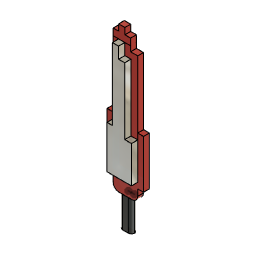
épée (Autodesk Fusion 360 design; units mm, degrees)
Autodesk Fusion 360 part; units mm, degrees
note: some values were not read from the file. Chosen so that the rebuilt part matches the saved one: which pieces of a blend or face edit are solid.
sketch "Esquisse1" plane through (0, 0, 0) normal (0, 0, 1) x (1, 0, 0)
  line L0 (304.8539, -213.5001) -> (-279.1145, -213.5001)
  line L1 (-279.1145, -213.5001) -> (-279.1145, 213.0938)
  line L2 (-279.1145, 213.0938) -> (304.8539, 213.0938)
  line L3 (304.8539, 213.0938) -> (304.8539, -213.5001)
  line L4 (443.4227, -65.0335) -> (-425, -65.0335)
  line L5 (-425, -65.0335) -> (-425, 75)
  line L6 (-425, 75) -> (443.4227, 75)
  line L7 (443.4227, 75) -> (443.4227, -65.0335)
  constraint horizontal L0
  constraint vertical L1
  constraint horizontal L2
  constraint vertical L3
  constraint horizontal L4
  constraint vertical L5
  constraint horizontal L6
  constraint vertical L7
extrude "Extrusion1" add sketch "Esquisse1" along normal blind 4200 makes body 1
sketch "Esquisse2" plane through (0, 213.0938, 0) normal (0, 1, 0) x (-1, 0, 0)
  line L0 (-304.8539, 0) -> (279.1145, 0)
  line L1 (279.1145, 0) -> (279.1145, 4200)
  line L2 (279.1145, 4200) -> (-304.8539, 4200)
  line L3 (-304.8539, 4200) -> (-304.8539, 0)
  line L4 (-304.8539, 1023.5422) -> (279.1145, 1023.5422)
  line L5 (279.1145, 1023.5422) -> (279.1145, 733.7125)
  line L6 (279.1145, 733.7125) -> (-304.8539, 733.7125)
  line L7 (-304.8539, 733.7125) -> (-304.8539, 1023.5422)
  line L8 (-12.8697, 733.7125) -> (-12.8697, 0)
  line L9 (131.0395, 733.7125) -> (-156.7789, 733.7125)
  line L10 (-156.7789, 733.7125) -> (-156.7789, 0)
  line L11 (-156.7789, 0) -> (131.0395, 0)
  line L12 (131.0395, 0) -> (131.0395, 733.7125)
  line L13 (131.0395, 733.7125) -> (-156.7789, 0) construction
  line L14 (-156.7789, 733.7125) -> (131.0395, 0) construction
  line L15 (-304.8539, 1023.5422) -> (-900, 1023.5422)
  line L16 (-900, 1023.5422) -> (-900, 0)
  line L17 (-900, 0) -> (-304.8539, 0)
  line L18 (-304.8539, 0) -> (-304.8539, 1023.5422)
  line L19 (-156.7789, 0) -> (-900, 0)
  line L20 (-900, 0) -> (-900, 733.7125)
  line L21 (-900, 733.7125) -> (-156.7789, 733.7125)
  line L22 (-156.7789, 733.7125) -> (-156.7789, 0)
  line L23 (279.1145, 1023.5422) -> (1050, 1023.5422)
  line L24 (1050, 1023.5422) -> (1050, 0)
  line L25 (1050, 0) -> (279.1145, 0)
  line L26 (279.1145, 0) -> (279.1145, 1023.5422)
  line L27 (131.0395, 733.7125) -> (1050, 733.7125)
  line L28 (1050, 733.7125) -> (1050, 0)
  line L29 (1050, 0) -> (131.0395, 0)
  line L30 (131.0395, 0) -> (131.0395, 733.7125)
  point P0 (-12.8697, 366.8562)
  constraint horizontal L4
  constraint vertical L5
  constraint horizontal L6
  constraint vertical L7
  constraint coincident L1 L5.end
  constraint coincident L3 L4.start
  constraint midpoint L6 L8.start
  constraint midpoint L0 L8.end
  constraint horizontal L9
  constraint perpendicular L9 L10
  constraint parallel L9 L11
  constraint parallel L10 L12
  constraint coincident L13 P0
  constraint coincident L14 P0
  constraint coincident L6 L9.start
  constraint midpoint L8 P0
  constraint horizontal L15
  constraint vertical L16
  constraint horizontal L17
  constraint vertical L18
  constraint horizontal L19
  constraint vertical L20
  constraint horizontal L21
  constraint vertical L22
  constraint coincident L16 L20.end
  constraint horizontal L23
  constraint vertical L24
  constraint horizontal L25
  constraint vertical L26
  constraint horizontal L27
  constraint vertical L28
  constraint horizontal L29
  constraint vertical L30
extrude "Extrusion2" cut sketch "Esquisse2" against normal blind 1050 contours L0 L3 L6 L10 L18 L19 L21 L22 | L3 L16 L17 L18 L19 L20 L21 | L3 L7 L15 L16 L18 L21 | L0 L1 L6 L12 L26 L27 L29 L30 | L1 L5 L23 L24 L26 L27 | L1 L24 L25 L26 L27 L28 L29 bodies 1
sketch "Esquisse3" plane through (0, 213.0938, 0) normal (0, 1, 0) x (-1, 0, 0)
  line L0 (-304.8539, 733.7125) -> (-156.7789, 733.7125)
  line L1 (-156.7789, 733.7125) -> (-156.7789, 0)
  line L2 (-156.7789, 0) -> (131.0395, 0)
  line L3 (131.0395, 0) -> (131.0395, 733.7125)
  line L4 (131.0395, 733.7125) -> (279.1145, 733.7125)
  line L5 (279.1145, 733.7125) -> (279.1145, 4200)
  line L6 (279.1145, 4200) -> (-304.8539, 4200)
  line L7 (-304.8539, 4200) -> (-304.8539, 733.7125)
  line L8 (-304.8539, 2175.6536) -> (-510, 2175.6536)
  line L9 (-510, 2175.6536) -> (-510, 4200)
  line L10 (-510, 4200) -> (-304.8539, 4200)
  line L11 (-304.8539, 4200) -> (-304.8539, 2175.6536)
  line L12 (279.1145, 2319.4912) -> (1100, 2319.4912)
  line L13 (1100, 2319.4912) -> (1100, 4400)
  line L14 (1100, 4400) -> (279.1145, 4400)
  line L15 (279.1145, 4400) -> (279.1145, 2319.4912)
  line L16 (150, 4050) -> (279.1145, 4050)
  line L17 (279.1145, 4050) -> (279.1145, 4400)
  line L18 (279.1145, 4400) -> (150, 4400)
  line L19 (150, 4400) -> (150, 4050)
  line L20 (0, 4050) -> (-304.8539, 4050)
  line L21 (-304.8539, 4050) -> (-304.8539, 4200)
  line L22 (-304.8539, 4200) -> (0, 4200)
  line L23 (0, 4200) -> (0, 4050)
  line L24 (-304.8539, 3767.2374) -> (-136.1037, 3767.2374)
  line L25 (-136.1037, 3767.2374) -> (-136.1037, 4050)
  line L26 (-136.1037, 4050) -> (-304.8539, 4050)
  line L27 (-304.8539, 4050) -> (-304.8539, 3767.2374)
  constraint horizontal L8
  constraint vertical L9
  constraint horizontal L10
  constraint vertical L11
  constraint coincident L7 L8.start
  constraint horizontal L12
  constraint vertical L13
  constraint horizontal L14
  constraint vertical L15
  constraint coincident L5 L12.start
  constraint horizontal L16
  constraint vertical L17
  constraint horizontal L18
  constraint vertical L19
  constraint horizontal L20
  constraint vertical L21
  constraint horizontal L22
  constraint vertical L23
  constraint coincident L6.end L7.start
  constraint horizontal L24
  constraint vertical L25
  constraint horizontal L26
  constraint vertical L27
  constraint coincident L20 L25.end
  constraint coincident L7 L24.start
extrude "Extrusion3" cut sketch "Esquisse3" against normal blind 1300 contours L7 L8 L9 L10 L11 L21 L27 | L7 L11 L20 L24 L25 L26 L27 | L6 L7 L11 L20 L21 L22 L23 L26 | L5 L12 L13 L14 L15 L17 | L6 L15 L17 L18 L19 | L5 L6 L15 L16 L17 L19 bodies 1
sketch "Esquisse4" plane through (-279.1145, 0, 0) normal (-1, 0, 0) x (0, -1, 0)
  line L0 (213.5001, 4050) -> (-213.0938, 4050)
  line L1 (-213.0938, 4050) -> (-213.0938, 733.7125)
  line L2 (-213.0938, 733.7125) -> (213.5001, 733.7125)
  line L3 (213.5001, 733.7125) -> (213.5001, 4050)
  line L4 (-75, 2319.4912) -> (65.0335, 2319.4912)
  line L5 (65.0335, 2319.4912) -> (65.0335, 1023.5422)
  line L6 (65.0335, 1023.5422) -> (-75, 1023.5422)
  line L7 (-75, 1023.5422) -> (-75, 2319.4912)
  line L8 (-75, 1023.5422) -> (-587.0309, 1023.5422)
  line L9 (-587.0309, 1023.5422) -> (-587.0309, -66.8511)
  line L10 (-587.0309, -66.8511) -> (-75, -66.8511)
  line L11 (-75, -66.8511) -> (-75, 1023.5422)
  line L12 (65.0335, 1023.5422) -> (650, 1023.5422)
  line L13 (650, 1023.5422) -> (650, -100)
  line L14 (650, -100) -> (65.0335, -100)
  line L15 (65.0335, -100) -> (65.0335, 1023.5422)
  line L16 (65.0335, 1023.5422) -> (340, 1023.5422)
  line L17 (340, 1023.5422) -> (340, 1160)
  line L18 (340, 1160) -> (65.0335, 1160)
  line L19 (65.0335, 1160) -> (65.0335, 1023.5422)
  line L20 (-75, 1023.5422) -> (-340, 1023.5422)
  line L21 (-340, 1023.5422) -> (-340, 1160)
  line L22 (-340, 1160) -> (-75, 1160)
  line L23 (-75, 1160) -> (-75, 1023.5422)
  constraint horizontal L8
  constraint vertical L9
  constraint horizontal L10
  constraint vertical L11
  constraint coincident L6.end L7.start
  constraint horizontal L12
  constraint vertical L13
  constraint horizontal L14
  constraint vertical L15
  constraint coincident L5.end L6.start
  constraint horizontal L16
  constraint vertical L17
  constraint horizontal L18
  constraint vertical L19
  constraint horizontal L20
  constraint vertical L21
  constraint horizontal L22
  constraint vertical L23
extrude "Extrusion4" cut sketch "Esquisse4" against normal blind 1600 contours L3 L12 L16 L17 L18 | L3 L5 L12 L16 L18 L19 | L1 L7 L8 L20 L22 L23 | L1 L8 L20 L21 L22 | L2 L3 L12 L13 L14 L15 L16 | L2 L3 L12 L15 L16 | L1 L2 L8 L11 L20 | L1 L2 L8 L9 L10 L11 L20 bodies 1
sketch "Esquisse5" plane through (-279.1145, 0, 0) normal (-1, 0, 0) x (0, -1, 0)
  line L0 (-213.0938, 1160) -> (-75, 1160)
  line L1 (-75, 1160) -> (-75, 2319.4912)
  line L2 (-75, 2319.4912) -> (65.0335, 2319.4912)
  line L3 (65.0335, 2319.4912) -> (65.0335, 1160)
  line L4 (65.0335, 1160) -> (213.5001, 1160)
  line L5 (213.5001, 1160) -> (213.5001, 4050)
  line L6 (213.5001, 4050) -> (-213.0938, 4050)
  line L7 (-213.0938, 4050) -> (-213.0938, 1160)
  line L8 (-70, 3890) -> (-364.9503, 3890)
  line L9 (-364.9503, 3890) -> (-364.9503, 4238.5385)
  line L10 (-364.9503, 4238.5385) -> (-70, 4238.5385)
  line L11 (-70, 4238.5385) -> (-70, 3890)
  line L12 (67.0373, 3890) -> (366.4832, 3890)
  line L13 (366.4832, 3890) -> (366.4832, 4314.6272)
  line L14 (366.4832, 4314.6272) -> (67.0373, 4314.6272)
  line L15 (67.0373, 4314.6272) -> (67.0373, 3890)
  constraint horizontal L8
  constraint vertical L9
  constraint horizontal L10
  constraint vertical L11
  constraint horizontal L12
  constraint vertical L13
  constraint horizontal L14
  constraint vertical L15
extrude "Extrusion5" cut sketch "Esquisse5" against normal blind 800 contours L6 L7 L8 L9 L10 L11 | L6 L7 L8 L11 | L5 L6 L12 L13 L14 L15 | L5 L6 L12 L15 bodies 1
sketch "Esquisse6" plane through (0, 213.0938, 0) normal (0, 1, 0) x (-1, 0, 0)
  line L0 (279.1145, 3890) -> (-136.1037, 3890)
  line L1 (-136.1037, 3890) -> (-136.1037, 3767.2374)
  line L2 (-136.1037, 3767.2374) -> (-304.8539, 3767.2374)
  line L3 (-304.8539, 3767.2374) -> (-304.8539, 1160)
  line L4 (-304.8539, 1160) -> (279.1145, 1160)
  line L5 (279.1145, 1160) -> (279.1145, 3890)
  line L6 (-144.0083, 2034.0359) -> (-304.8539, 2034.0359)
  line L7 (-304.8539, 2034.0359) -> (-304.8539, 3767.2374)
  line L8 (-304.8539, 3767.2374) -> (-144.0083, 3767.2374)
  line L9 (-144.0083, 3767.2374) -> (-144.0083, 2034.0359)
  line L10 (2.2284, 3618.7555) -> (-136.1037, 3618.7555)
  line L11 (-136.1037, 3618.7555) -> (-136.1037, 3890)
  line L12 (-136.1037, 3890) -> (2.2284, 3890)
  line L13 (2.2284, 3890) -> (2.2284, 3618.7555)
  line L14 (148.5698, 3890) -> (279.1145, 3890)
  line L15 (279.1145, 3890) -> (279.1145, 2179.5393)
  line L16 (279.1145, 2179.5393) -> (148.5698, 2179.5393)
  line L17 (148.5698, 2179.5393) -> (148.5698, 3890)
  constraint horizontal L6
  constraint vertical L7
  constraint horizontal L8
  constraint vertical L9
  constraint coincident L2.end L3.start
  constraint horizontal L10
  constraint vertical L11
  constraint horizontal L12
  constraint vertical L13
  constraint coincident L0.end L1.start
  constraint horizontal L14
  constraint vertical L15
  constraint horizontal L16
  constraint vertical L17
  constraint coincident L5 L15.end
  constraint coincident L0 L14.start
extrude "Extrusion6" cut sketch "Esquisse6" against normal blind 140 contours L0 L5 L14 L15 L16 L17 | L0 L1 L10 L11 L12 L13 | L2 L3 L6 L7 L8 L9 bodies 1
sketch "Esquisse7" plane through (0, -213.5001, 0) normal (0, -1, 0) x (1, 0, 0)
  line L0 (136.1037, 3890) -> (-279.1145, 3890)
  line L1 (-279.1145, 3890) -> (-279.1145, 1160)
  line L2 (-279.1145, 1160) -> (304.8539, 1160)
  line L3 (304.8539, 1160) -> (304.8539, 3767.2374)
  line L4 (304.8539, 3767.2374) -> (136.1037, 3767.2374)
  line L5 (136.1037, 3767.2374) -> (136.1037, 3890)
  line L6 (-150, 2175) -> (-279.1145, 2175)
  line L7 (-279.1145, 2175) -> (-279.1145, 3890)
  line L8 (-279.1145, 3890) -> (-150, 3890)
  line L9 (-150, 3890) -> (-150, 2175)
  line L10 (-2.9663, 3890) -> (138.4468, 3890)
  line L11 (138.4468, 3890) -> (138.4468, 3621.153)
  line L12 (138.4468, 3621.153) -> (-2.9663, 3621.153)
  line L13 (-2.9663, 3621.153) -> (-2.9663, 3890)
  line L14 (136.1037, 3767.2374) -> (304.8539, 3767.2374)
  line L15 (304.8539, 3767.2374) -> (304.8539, 2032.7398)
  line L16 (304.8539, 2032.7398) -> (136.1037, 2032.7398)
  line L17 (136.1037, 2032.7398) -> (136.1037, 3767.2374)
  constraint horizontal L6
  constraint vertical L7
  constraint horizontal L8
  constraint vertical L9
  constraint coincident L0.end L1.start
  constraint horizontal L10
  constraint vertical L11
  constraint horizontal L12
  constraint vertical L13
  constraint coincident L0 L10.start
  constraint horizontal L14
  constraint vertical L15
  constraint horizontal L16
  constraint vertical L17
  constraint coincident L3 L15.end
  constraint coincident L4.end L5.start
extrude "Extrusion7" cut sketch "Esquisse7" against normal blind 140 contours L0 L5 L10 L12 L13 L17 | L0 L1 L6 L7 L8 L9 | L3 L4 L11 L12 L14 L15 L16 L17 bodies 1
sketch "Esquisse8" plane through (136.1037, 0, 0) normal (-1, 0, 0) x (0, -1, 0)
  line L0 (-73.0938, 3767.2374) -> (-213.0938, 3767.2374)
  line L1 (-213.0938, 3767.2374) -> (-213.0938, 3618.7555)
  line L2 (-213.0938, 3618.7555) -> (-73.0938, 3618.7555)
  line L3 (-73.0938, 3618.7555) -> (-73.0938, 3767.2374)
  line L4 (-73.0938, 3618.7555) -> (-213.0938, 3618.7555)
  line L5 (-213.0938, 3618.7555) -> (-213.0938, 3767.2374)
  line L6 (-213.0938, 3767.2374) -> (-73.0938, 3767.2374)
  line L7 (-73.0938, 3767.2374) -> (-73.0938, 3618.7555)
  constraint horizontal L4
  constraint vertical L5
  constraint horizontal L6
  constraint vertical L7
  constraint coincident L0.end L1.start
  constraint coincident L2.end L3.start
extrude "Extrusion8" cut sketch "Esquisse8" against normal blind 350 bodies 1
sketch "Esquisse9" plane through (136.1037, 0, 0) normal (-1, 0, 0) x (0, -1, 0)
  line L0 (213.5001, 3767.2374) -> (73.5001, 3767.2374)
  line L1 (73.5001, 3767.2374) -> (73.5001, 3621.153)
  line L2 (73.5001, 3621.153) -> (213.5001, 3621.153)
  line L3 (213.5001, 3621.153) -> (213.5001, 3767.2374)
  line L4 (73.5001, 3621.153) -> (213.5001, 3621.153)
  line L5 (213.5001, 3621.153) -> (213.5001, 3767.2374)
  line L6 (213.5001, 3767.2374) -> (73.5001, 3767.2374)
  line L7 (73.5001, 3767.2374) -> (73.5001, 3621.153)
  constraint horizontal L4
  constraint vertical L5
  constraint horizontal L6
  constraint vertical L7
  constraint coincident L0.start L3.end
  constraint coincident L1.end L2.start
extrude "Extrusion9" cut sketch "Esquisse9" against normal blind 150 bodies 1
extrude "Extrusion10" add 1 faces at (-47.6703, -67.0373, 3943.3333) along direction (0, -1, 0) blind 6.5 on bodies 1 bodies 1
extrude "Extrusion11" add 1 faces at (-47.6703, 70, 3943.3333) along direction (0, 1, 0) blind 3.1 on bodies 1 bodies 1
fillet "Congé1" radius 75 4 edges at (-131.0395, -65.0335, 366.8562) (156.7789, -65.0335, 366.8562) (-131.0395, 75, 366.8562) (156.7789, 75, 366.8562) on bodies 1
fillet "Congé2" radius 137.5 2 edges at (-279.1145, 4.9832, 733.7125) (304.8539, 4.9832, 733.7125) on bodies 1
extrude "Extrusion12" cut 1 faces at (-236.0764, -73.5001, 3318.3333) along direction (0, 1, 0) blind 8.4666 on bodies 1 bodies 1
extrude "Extrusion13" cut 1 faces at (-50.9888, -73.5373, 3996.6667) along direction (0, 1, 0) blind 8.5 on bodies 1 bodies 1
extrude "Extrusion14" cut 1 faces at (248.6038, -73.5001, 3140.3767) along direction (0, 1, 0) blind 8.5 on bodies 1 bodies 1
extrude "Extrusion15" add 1 faces at (56.5826, 213.0938, 1451.3453) along direction (0, -1, 0) blind 426.594 separate body on bodies 1 makes body 2
extrude "Extrusion16" cut 1 faces at (56.5826, 213.0938, 1451.3453) along direction (0, -1, 0) blind 1600 on bodies 1 bodies 1
sketch "Esquisse10" plane through (0, 75, 0) normal (0, 1, 0) x (-1, 0, 0)
  arc A0 (-304.8539, 871.2125) -> (-167.3539, 733.7125) centre (-167.3539, 871.2125) ccw
  line L0 (-167.3539, 733.7125) -> (-82.444, 733.7125)
  line L1 (-82.444, 733.7125) -> (-82.444, 0)
  line L2 (-82.444, 0) -> (56.7047, 0)
  line L3 (56.7047, 0) -> (56.7047, 733.7125)
  line L4 (56.7047, 733.7125) -> (141.6145, 733.7125)
  arc A1 (141.6145, 733.7125) -> (279.1145, 871.2125) centre (141.6145, 871.2125) ccw
  line L5 (279.1145, 871.2125) -> (279.1145, 1023.5422)
  line L6 (279.1145, 1023.5422) -> (425, 1023.5422)
  line L7 (425, 1023.5422) -> (425, 2319.4912)
  line L8 (425, 2319.4912) -> (279.1145, 2319.4912)
  line L9 (279.1145, 2319.4912) -> (279.1145, 1160)
  line L10 (279.1145, 1160) -> (-304.8539, 1160)
  line L11 (-304.8539, 1160) -> (-304.8539, 2175.6536)
  line L12 (-304.8539, 2175.6536) -> (-443.4227, 2175.6536)
  line L13 (-443.4227, 2175.6536) -> (-443.4227, 1023.5422)
  line L14 (-443.4227, 1023.5422) -> (-304.8539, 1023.5422)
  line L15 (-304.8539, 1023.5422) -> (-304.8539, 871.2125)
  line L16 (-82.444, 733.7125) -> (56.7047, 733.7125)
  constraint coincident L0.end L1.start
  constraint coincident L3.end L4.start
sketch "Esquisse11" plane through (0, -65.0335, 0) normal (0, -1, 0) x (1, 0, 0)
  arc A0 (167.3539, 733.7125) -> (304.8539, 871.2125) centre (167.3539, 871.2125) ccw
  line L0 (304.8539, 871.2125) -> (304.8539, 1023.5422)
  line L1 (304.8539, 1023.5422) -> (443.4227, 1023.5422)
  line L2 (443.4227, 1023.5422) -> (443.4227, 2175.6536)
  line L3 (443.4227, 2175.6536) -> (304.8539, 2175.6536)
  line L4 (304.8539, 2175.6536) -> (304.8539, 1160)
  line L5 (304.8539, 1160) -> (-279.1145, 1160)
  line L6 (-279.1145, 1160) -> (-279.1145, 2319.4912)
  line L7 (-279.1145, 2319.4912) -> (-425, 2319.4912)
  line L8 (-425, 2319.4912) -> (-425, 1023.5422)
  line L9 (-425, 1023.5422) -> (-279.1145, 1023.5422)
  line L10 (-279.1145, 1023.5422) -> (-279.1145, 871.2125)
  arc A1 (-279.1145, 871.2125) -> (-141.6145, 733.7125) centre (-141.6145, 871.2125) ccw
  line L11 (-141.6145, 733.7125) -> (-56.0395, 733.7125)
  line L12 (-56.0395, 733.7125) -> (-56.0395, 0)
  line L13 (-56.0395, 0) -> (81.7789, 0)
  line L14 (81.7789, 0) -> (81.7789, 733.7125)
  line L15 (81.7789, 733.7125) -> (167.3539, 733.7125)
  line L16 (-56.0395, 733.7125) -> (81.7789, 733.7125)
  constraint coincident L11.end L12.start
  constraint coincident L14.end L15.start
split "Scinder1" by curves path "Esquisse11" along L16 bodies 1 makes body 3 at (-10.1, 75, 244.5708)
extrude "Extrusion17" cut 1 faces at (43.8823, -164.0001, 3621.153) along direction (0, 0, -1) blind 100 on bodies 1 bodies 1
extrude "Extrusion18" cut 1 faces at (-150, -114.5236, 2749.6929) along direction (1, 0, 0) blind 1200 on bodies 1 bodies 1
